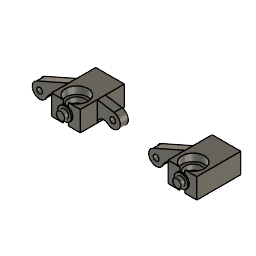
Steering knuckle2 (Autodesk Fusion 360 design; units mm, degrees)
Autodesk Fusion 360 part; units mm, degrees
sketch "Skizze1" plane through (0, 0, 0) normal (0, 0, 1) x (1, 0, 0)
  circle A0 centre (0, 0) radius 4.1
  circle A1 centre (0, 0) radius 3.05
  circle A2 centre (0, 0) radius 5.35
  dimension "d1" = 8.2
  dimension "d2" = 6.1
  dimension "d3" = 10.7
  constraint coincident A0.centre A1.centre
  constraint concentric A0 A1
  measures "d1" diameter of A0
  measures "d2" diameter of A1
  measures "d3" diameter of A2
sketch "Skizze2" plane through (0, 0, 0) normal (0, 1, 0) x (1, 0, 0)
  line L0 (5.3, -3.75) -> (-5.3, -3.75)
  line L1 (-5.3, -3.75) -> (-5.3, 3.75)
  line L2 (-5.3, 3.75) -> (5.3, 3.75)
  line L3 (5.3, 3.75) -> (5.3, -3.75)
  dimension "d41" = 7.5
  dimension "d44" = 3.75
  dimension "d46" = 10.6
  dimension "d47" = 5.3
  constraint horizontal L0
  constraint vertical L1
  constraint horizontal L2
  constraint vertical L3
  measures "d41" distance of L0 L2
  measures "d44" distance of L0 origin
  measures "d46" distance of L1 L3
  measures "d47" distance of L1 origin
extrude "Extrusion7" add sketch "Skizze2" along normal blind 5.3 makes body 1
extrude "Extrusion8" add sketch "Skizze2" against normal blind 5.3 bodies 1
extrude "Extrusion9" cut sketch "Skizze1" against normal blind 20 from surface at 10 contours A1 bodies 1
extrude "Extrusion10" cut sketch "Skizze1" against normal blind 10 from surface at -1 contours A0 bodies 1
extrude "Extrusion11" cut sketch "Skizze1" along normal blind 10 from surface at 1 contours A0 bodies 1
sketch "Skizze4" plane through (0, 5.3, 0) normal (0, 1, 0) x (-1, 0, 0)
  line L0 (-5.3, -3.75) -> (5.3, -3.75)
  line L1 (5.3, -3.75) -> (5.3, 3.75)
  line L2 (5.3, 3.75) -> (-5.3, 3.75)
  line L3 (-5.3, 3.75) -> (-5.3, -3.75)
  circle A0 centre (0, 0) radius 1.525
  circle A1 centre (0, 0) radius 2.525
  line L4 (5.3, -4.9263) -> (5.3, 3.75)
  circle A2 centre (16, -4) radius 2.7645
  circle A3 centre (16, -4) radius 1.05
  line L5 (5.3, 3.75) -> (17.1173, -1.4714)
  circle A4 centre (-11, 0) radius 1.05
  circle A5 centre (-11, 0) radius 2.7645
  line L6 (-5.3, 3.75) -> (-11.4534, 2.7271)
  arc A6 (-5.3, -3.75) -> (-9.1532, -2.0571) centre (-7.6099, -3.776) ccw
  arc A7 (13.574, -5.3255) -> (5.3, -3.75) centre (8.9254, -7.2244) ccw
  dimension "d45" = 3.05
  dimension "d56" = 5.05
  dimension "d65" = 7.5
  dimension "d66" = 2.1
  dimension "d67" = 5.529
  dimension "d91" = 16
  dimension "d92" = 16
  dimension "d95" = 3.75
  dimension "d102" = 2.1
  dimension "d103" = 5.529
  dimension "d104" = 11
  dimension "d110" = 7.75
  dimension "d111" = 3.75
  constraint coincident A0.centre A1.centre
  constraint concentric A0 A1
  constraint vertical L4
  constraint collinear L1 L4
  constraint concentric A2 A3
  constraint coincident A2 L5.end
  constraint tangent A2 L5
  constraint coincident L1.end L2.start
  constraint concentric A4 A5
  constraint coincident L2.end L3.start
  constraint coincident A5 L6.end
  constraint tangent A5 L6
  constraint tangent A5 A6
  constraint coincident A5 A6.end
  constraint coincident L0.start L3.end
  constraint coincident L0.end L1.start
  constraint coincident A2 A7.start
  measures "d45" diameter of A0
  measures "d56" diameter of A1
  measures "d65" distance of L0 L2
  measures "d66" diameter of A3
  measures "d67" diameter of A2
  measures "d91" horizontal distance of A0.centre A2.centre
  measures "d92" horizontal distance of A0.centre A2.centre
  measures "d95" distance of L0 A0.centre
  measures "d102" diameter of A4
  measures "d103" diameter of A5
  measures "d104" horizontal distance of A0.centre A4.centre
  measures "d110" distance of L2 A2.centre
  measures "d111" distance of L2 A4.centre
extrude "Extrusion16" cut sketch "Skizze2" against normal blind 4.2 from surface at -4 bodies 1
extrude "Extrusion17" add sketch "Skizze4" against normal blind 2 from surface at -9.3 contours A0 bodies 1
extrude "Extrusion20" add sketch "Skizze4" against normal blind 3 contours L1 L4 A2 L5 A7 bodies 1
extrude "Extrusion21" add sketch "Skizze4" against normal blind 0.5 from surface at -9.3 contours A1 bodies 1
extrude "Extrusion32" add sketch "Skizze4" along normal blind 7 contours L0 L1 L2 L3 L4 | A0 | A1 bodies 1
extrude "Extrusion26" add sketch "Skizze4" against normal blind 3 contours L1 L4 A2 L5 A7 | A2 A7 | A2 A7 bodies 1
extrude "Extrusion34" add sketch "Skizze4" along normal blind 0.5 from surface at 7 contours A1 bodies 1
extrude "Extrusion35" add sketch "Skizze4" along normal blind 2 from surface at 7 contours A0 bodies 1
pattern_linear "R-Anordnung1" count 2 spacing 43 along (1, 0, 0) of bodies 1 makes body 2
extrude "Extrusion30" add sketch "Skizze4" against normal blind 3 contours L3 A5 L6 A6 | A5 bodies 1
equation "d3 = d1 + 2.5 mm"
equation "d41 = 5 mm + 2 mm + 0.5 mm"
equation "d44 = d41 / 2"
equation "d47 = d46 / 2"
equation "d56 = d45 + 2 mm"
equation "d67 = d68"
equation "d68 = 5.5289569917 mm"
equation "d69 = d67 / 2"
equation "d102 = d66"
equation "d103 = d67"
equation "d110 = 4 mm + d95"
equation "d111 = d95"
